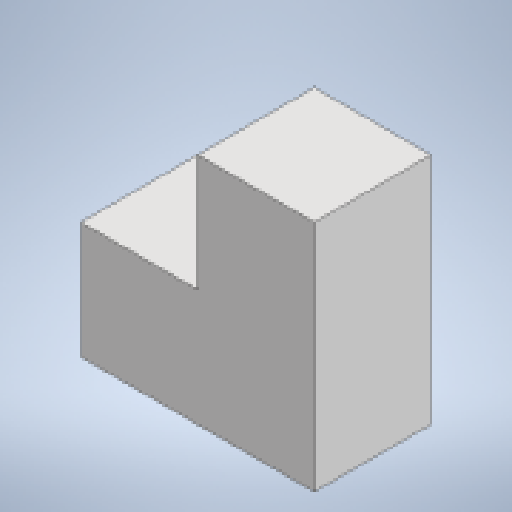
# Autodesk Inventor part: chest_box_cap_connect
Saved by Autodesk Inventor 2024 (Build 280153000, 153)
## iProperties
Created: 2024-09-18
Part Number: chest_box_cap_connect
Material: 일반
Document SubType Name: Modeling
Designer: Eungang
Density: 1 g/cm^3
Appearance: 기본값
Author: Eungang
Autodesk Inventor part; units mm, degrees
ref_plane "YZ Plane" through (0, 0, 0) normal (1, 0, 0) x (0, 1, 0)
ref_plane "XZ Plane" through (0, 0, 0) normal (0, 1, 0) x (-1, 0, 0)
ref_plane "XY Plane" through (0, 0, 0) normal (0, 0, 1) x (1, 0, 0)
sketch "스케치1" plane through (0, 0, 0) normal (0, 0, 1) x (1, 0, 0)
  line L0 (-71.3, 53.4) -> (-71.3, -53.4) projected
  line L1 (-71.3, -53.4) -> (71.3, -53.4) projected
  line L2 (71.3, -53.4) -> (71.3, 53.4) projected
  line L3 (71.3, 53.4) -> (-71.3, 53.4) projected
  line L4 (71.3, -53.4) -> (59.3, -53.4)
  line L5 (59.3, -53.4) -> (59.3, -47.4)
  line L6 (59.3, -47.4) -> (71.3, -47.4)
  line L7 (71.3, -47.4) -> (71.3, -53.4)
  line L8 (71.3, -53.4) -> (65.3, -53.4)
  line L9 (65.3, -53.4) -> (65.3, -41.4)
  line L10 (65.3, -41.4) -> (71.3, -41.4)
  line L11 (71.3, -41.4) -> (71.3, -53.4)
  circle A0 centre (68.3, -50.4) radius 1.35
  circle A1 centre (68.3, 50.4) radius 1.35 projected
  circle A2 centre (-68.3, 50.4) radius 1.35 projected
  circle A3 centre (-68.3, -50.4) radius 1.35 projected
  circle A4 centre (68.3, -50.4) radius 1.35 projected
  point P0 (0, 0)
  point P1 (65.3, -47.4)
  dimension "d0" = 12
  dimension "d1" = 6
  dimension "d2" = 6
  dimension "d3" = 12
  dimension "d12" = 2.7
  constraints: 16 end point, 4 parallel, 2 horizontal, 2 perpendicular, 1 centre point
  measures "d0" distance of L5.end L6.end
  measures "d1" distance of L4.end L5.end
  measures "d2" distance of L9.end L10.end
  measures "d3" distance of L8.end L9.end
  measures "d12" diameter of A0
extrude "돌출1" add sketch "스케치1" along normal blind 6 contours L5 L6 L9 L1 | L2 L6 L9 L10 | L9 L6 L2 L1
sketch "스케치2" plane through (59.3, -47.4, 0) normal (0, 1, 0) x (1, 0, 0)
  line L0 (0, 0) -> (0, -6) projected
  line L1 (0, -3) -> (6, -3)
  line L2 (6, 0) -> (6, -6) projected
  circle A0 centre (3, -3) radius 1.35
  point P0 (-59.3, 0)
  dimension "d6" = 2.7
  constraints: 3 midpoint, 2 end point, 1 centre point
  measures "d6" diameter of A0
extrude "돌출2" cut sketch "스케치2" against normal up to next
sketch "스케치3" plane through (65.3, -47.4, 0) normal (-1, 0, 0) x (0, 0, 1)
  line L0 (0, 6) -> (0, 0) projected
  line L1 (0, 0) -> (6, 0) projected
  line L2 (6, 6) -> (6, 0) projected
  line L3 (0, 6) -> (6, 6) projected
  circle A0 centre (3, 3) radius 1.35
  point P0 (0, 47.4)
  dimension "d9" = 2.7
  constraints: 1 centre point
  measures "d9" diameter of A0
extrude "돌출3" cut sketch "스케치3" against normal up to next contours A0
